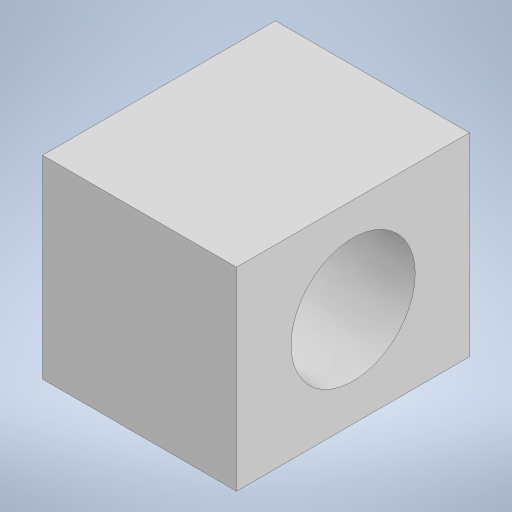
# Autodesk Inventor part: lcdholder
Saved by Autodesk Inventor 2023 (Build 270158000, 158)
## iProperties
Created: 2025-09-11
Part Number: lcdholder
Material: Generic
Document SubType Name: Modeling
Designer: ptato_qo49uko
Density: 1 g/cm^3
Appearance: Default
Author: ptato_qo49uko
Autodesk Inventor part; units mm, degrees
ref_plane "YZ Plane" through (0, 0, 0) normal (1, 0, 0) x (0, 1, 0)
ref_plane "XZ Plane" through (0, 0, 0) normal (0, 1, 0) x (-1, 0, 0)
ref_plane "XY Plane" through (0, 0, 0) normal (0, 0, 1) x (1, 0, 0)
sketch "Sketch1" plane through (0, 0, 0) normal (1, 0, 0) x (0, 1, 0)
  line L0 (22.8278, 24.0961) -> (17.8278, 24.0961)
  line L1 (17.8278, 24.0961) -> (17.8278, 18.0961)
  line L2 (17.8278, 18.0961) -> (22.8278, 18.0961)
  line L3 (22.8278, 18.0961) -> (22.8278, 24.0961)
  point P0 (0, 0)
  dimension "d0" = 5
  dimension "d1" = 6
  constraints: 8 end point, 2 parallel, 1 horizontal, 1 perpendicular
  measures "d0" distance of L2.end L1.end
  measures "d1" distance of L1.end L0.end
extrude "Extrusion1" add sketch "Sketch1" along normal blind 5
sketch "Sketch2" plane through (5, 0, 0) normal (1, 0, 0) x (0, 0, -1)
  point P0 (0, 0)
  point P1 (-21.0928, 20.384)
hole "Hole1" at (5, 20.384, 21.0928) direction (-1, 0, 0) diameter 3.2 end through all
body "Solid1"
